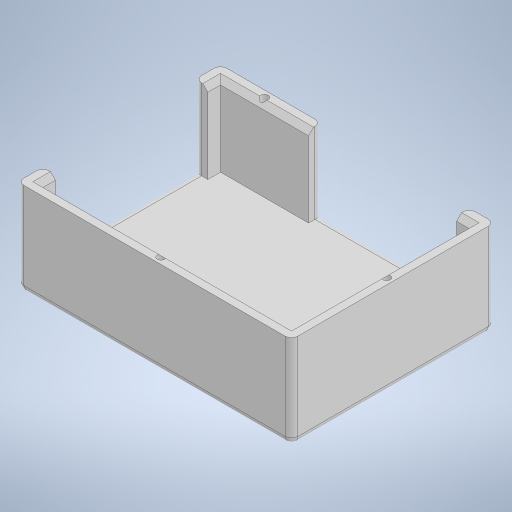
# Autodesk Inventor part: housing_bottom
Saved by Autodesk Inventor 2024 (Build 280153000, 153)
## iProperties
Created: 2024-03-11
Part Number: housing_bottom
Material: 일반
Document SubType Name: Modeling
Designer: SSAFY
Density: 1 g/cm^3
Appearance: 기본값
Author: SSAFY
Autodesk Inventor part; units mm, degrees
ref_plane "YZ Plane" through (0, 0, 0) normal (1, 0, 0) x (0, 1, 0)
ref_plane "XZ Plane" through (0, 0, 0) normal (0, 1, 0) x (-1, 0, 0)
ref_plane "XY Plane" through (0, 0, 0) normal (0, 0, 1) x (1, 0, 0)
sketch "스케치2" plane through (0, 0, 0) normal (0, 1, 0) x (-1, 0, 0)
  line L0 (-49.375, 35.275) -> (49.375, 35.275)
  line L1 (49.375, 35.275) -> (49.375, -35.275)
  line L2 (49.375, -35.275) -> (-49.375, -35.275)
  line L3 (-49.375, -35.275) -> (-49.375, 35.275)
  line L4 (-49.375, 35.275) -> (49.375, -35.275) construction
  line L5 (49.375, 35.275) -> (-49.375, -35.275) construction
  line L6 (-54.375, -40.275) -> (54.375, -40.275)
  line L7 (54.375, -40.275) -> (54.375, 40.275)
  line L8 (54.375, 40.275) -> (-54.375, 40.275)
  line L9 (-54.375, 40.275) -> (-54.375, -40.275)
  point P0 (0, 0)
  dimension "d0" = 98.75
  dimension "d1" = 70.55
  dimension "d2" = 5
  constraints: 20 end point, 4 parallel, 2 midpoint, 2 perpendicular, 1 horizontal, 3 other
  measures "d0" distance of L1.end L2.end
  measures "d1" distance of L2.end L0.start
  measures "d2" distance between parallel lines of L1 L7
extrude "돌출1" add sketch "스케치2" along normal blind 32
sketch "스케치3" plane through (0, 0, 0) normal (0, 1, 0) x (-1, 0, 0)
  line L0 (-54.375, 40.275) -> (-54.375, -40.275) construction
  line L1 (54.375, -40.275) -> (-54.375, -40.275)
  line L2 (-54.375, -40.275) -> (-54.375, 40.275)
  line L3 (-54.375, 40.275) -> (54.375, 40.275)
  line L4 (54.375, 40.275) -> (54.375, -40.275)
  line L5 (54.375, -40.275) -> (-54.375, 40.275) construction
  line L6 (-54.375, -40.275) -> (54.375, 40.275) construction
  point P0 (0, 0)
  constraints: 12 end point, 2 midpoint, 2 parallel, 1 horizontal, 1 perpendicular
extrude "돌출2" add sketch "스케치3" against normal blind 5
sketch "스케치4" plane through (0, 0, 0) normal (0, 1, 0) x (-1, 0, 0)
  line L0 (49.375, 35.275) -> (49.375, -35.275) construction
  line L1 (54.375, -40.275) -> (54.375, 40.275) construction
  line L2 (49.375, 30.275) -> (54.375, 30.275)
  line L3 (54.375, 30.275) -> (54.375, -30.275)
  line L4 (54.375, -30.275) -> (49.375, -30.275)
  line L5 (49.375, -30.275) -> (49.375, 30.275)
  line L6 (-49.375, 35.275) -> (49.375, 35.275) construction
  line L7 (49.375, -35.275) -> (-49.375, -35.275) construction
  line L8 (54.375, -40.275) -> (-54.375, -40.275) construction
  line L9 (-44.375, -35.275) -> (14.375, -35.275)
  line L10 (14.375, -35.275) -> (14.375, -40.275)
  line L11 (14.375, -40.275) -> (-44.375, -40.275)
  line L12 (-44.375, -40.275) -> (-44.375, -35.275)
  line L13 (-49.375, -35.275) -> (-49.375, 35.275) construction
  point P0 (0, 0)
  dimension "d7" = 5
  dimension "d8" = 5
  dimension "d11" = 5
  dimension "d12" = 35
  constraints: 16 end point, 4 parallel, 4 point on line, 2 horizontal, 2 perpendicular
  measures "d7" distance between parallel lines of L6 L2
  measures "d8" distance between parallel lines of L7 L4
  measures "d11" distance between parallel lines of L13 L12
  measures "d12" distance between parallel lines of L0 L10
extrude "돌출3" cut sketch "스케치4" along normal through all
sketch "스케치5" plane through (0, 32, 0) normal (0, 1, 0) x (1, 0, 0)
  line L0 (49.375, 35.275) -> (49.375, -35.275) construction
  line L1 (49.375, -35.275) -> (-49.375, -35.275) construction
  circle A0 centre (0, -37.775) radius 1.5
  circle A1 centre (51.875, 0) radius 1.5
  circle A2 centre (-34.375, 37.775) radius 1.5
  line L2 (-49.375, 35.275) -> (-14.375, 35.275) construction
  line L3 (-54.375, 40.275) -> (-54.375, 30.275) construction
  point P0 (0, 0)
  dimension "d17" = 3
  dimension "d18" = 2.5
  dimension "d19" = 3
  dimension "d20" = 2.5
  dimension "d21" = 3
  dimension "d22" = 2.5
  dimension "d23" = 20
  constraints: 3 centre point
  measures "d17" diameter of A0
  measures "d18" distance from line of L1 A0.centre
  measures "d19" diameter of A1
  measures "d20" distance from line of A1.centre L0
  measures "d21" diameter of A2
  measures "d22" distance from line of A2.centre L2
  measures "d23" distance from line of L3 A2.centre
extrude "돌출4" cut sketch "스케치5" against normal blind 5
fillet "모깎기1" radius 2.5 14 edges at (-54.375, 13.5, 40.275) (54.375, 13.5, 40.275) (54.375, 13.5, -40.275) (-54.375, 13.5, -40.275) (-54.375, -5, 0) (0, -5, -40.275) (0, -5, 40.275) (54.375, -5, 0) (-14.375, 16, -40.275) (15, 0, -40.275) (44.375, 16, -40.275) (-54.375, 16, 30.275) (-54.375, 0, 0) (-54.375, 16, -30.275)
chamfer "모따기1" distance 2 angle 45 6 edges at (-31.875, 32, -35.275) (-49.375, 32, -32.775) (-49.375, 32, 32.775) (0, 32, 35.275) (49.375, 32, 0) (46.875, 32, -35.275)
